rod_end_cap (Autodesk Fusion 360 design; units mm, degrees)
part number: 2026-09-03-23-52-10-226
Autodesk Fusion 360 part; units mm, degrees
sketch "End cap profile" plane through (0, 0, 0) normal (0, 1, 0) x (1, 0, 0)
  line L0 (0, 0) -> (21, 0)
  line L1 (21, 0) -> (21, -4)
  line L2 (21, -4) -> (14.7, -4)
  line L3 (14.7, -4) -> (14.7, -25.5)
  line L4 (14.7, -25.5) -> (12.2, -28)
  line L5 (12.2, -28) -> (0, -28)
  line L6 (0, -28) -> (0, 0)
  dimension "d60" = 21
  dimension "d61" = 4
  dimension "d62" = 14.7
  dimension "d63" = 28
  dimension "d64" = 2.5
  dimension "d65" = 2.5
  constraint horizontal L0
  constraint horizontal L2
  constraint horizontal L5
  constraint vertical L1
  constraint vertical L3
  constraint vertical L6
  constraint coincident L0.start L6.end
  measures "d60" horizontal distance of L0.start L0.end
  measures "d61" vertical distance of L0.end L1.end
  measures "d62" horizontal distance of L0.start L2.end
  measures "d63" vertical distance of L0.start L5.end
  measures "d64" horizontal distance of L3.end L4.end
  measures "d65" vertical distance of L3.end L4.end
revolve "End cap revolve" add sketch "End cap profile" angle 360 about axis through (0, 0, 1.75) along (0, 0, 1)
sketch "Crush rib" plane through (0, 0, 0) normal (0, 1, 0) x (1, 0, 0)
  line L0 (13.7, -5) -> (15.2, -5)
  line L1 (15.2, -5) -> (15.2, -11)
  line L2 (15.2, -11) -> (13.7, -26)
  line L3 (13.7, -26) -> (13.7, -5)
  dimension "d67" = 13.7
  dimension "d68" = 5
  dimension "d69" = 15.2
  dimension "d70" = 26
  dimension "d71" = 11
  constraint horizontal L0
  constraint vertical L1
  constraint vertical L3
  measures "d67" horizontal distance of origin L0.start
  measures "d68" vertical distance of origin L0.start
  measures "d69" horizontal distance of origin L0.end
  measures "d70" vertical distance of origin L2.end
  measures "d71" vertical distance of origin L1.end
extrude "Crush rib (1)" add sketch "Crush rib" along normal mid plane 2
pattern_circular "Crush ribs" count 4 over 360 about axis through (0, 0, 1.75) along (0, 0, 1) of "Crush rib (1)"
equation "rodOuterDiameter = 33.4 mm" comment "drives the model; safe to edit live in Fusion"
equation "pipeInnerDiameter = 30.0 mm" comment "drives the model; safe to edit live in Fusion"
equation "endCapFlangeProud = 4.3 mm" comment "drives the model; safe to edit live in Fusion"
equation "endCapFlangeThickness = 4.0 mm" comment "drives the model; safe to edit live in Fusion"
equation "endCapStemLength = 24.0 mm" comment "drives the model; safe to edit live in Fusion"
equation "endCapStemDiameter = pipeInnerDiameter - 0.6 mm" comment "drives the model; safe to edit live in Fusion"
equation "endCapRibDiameter = pipeInnerDiameter + 0.4 mm" comment "drives the model; safe to edit live in Fusion"
equation "endCapTipChamfer = 2.5 mm" comment "drives the model; safe to edit live in Fusion"
equation "endCapRibWidth = 2.0 mm" comment "drives the model; safe to edit live in Fusion"
equation "endCapRibCount = 4" comment "drives the model; safe to edit live in Fusion"
equation "endCapRibGripLength = 6.0 mm" comment "drives the model; safe to edit live in Fusion"
equation "d60 = rodOuterDiameter / 2 + endCapFlangeProud"
equation "d61 = endCapFlangeThickness"
equation "d62 = endCapStemDiameter / 2"
equation "d63 = endCapFlangeThickness + endCapStemLength"
equation "d64 = endCapTipChamfer"
equation "d65 = endCapTipChamfer"
equation "d67 = endCapStemDiameter / 2 - 1 mm"
equation "d68 = endCapFlangeThickness + 1 mm"
equation "d69 = endCapRibDiameter / 2"
equation "d70 = endCapFlangeThickness + endCapStemLength - 2 mm"
equation "d71 = endCapFlangeThickness + 1 mm + endCapRibGripLength"
equation "d72 = endCapRibWidth"
equation "d74 = endCapRibCount"
named bodies: "rod_end_cap"
